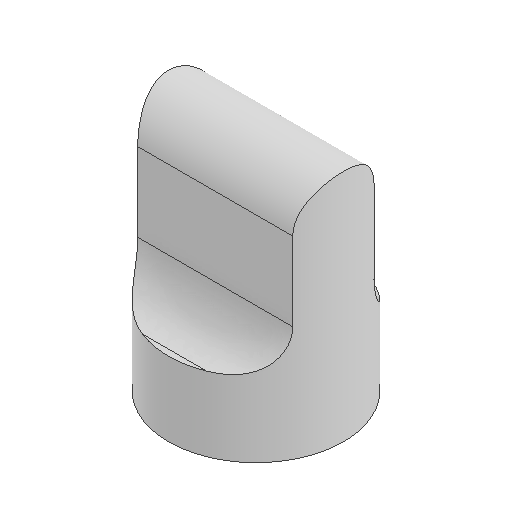
# Autodesk Inventor part: Half Universal
Saved by Autodesk Inventor 2025 (Build 290162010, 162A)
## iProperties
Created: 2024-12-02
Part Number: Half Universal
Material: Generic
Document SubType Name: Modeling
Designer: ALEXANDERNICHOLS
Density: 1 g/cm^3
Appearance: Default
Author: ALEXANDERNICHOLS
Autodesk Inventor part; units mm, degrees
ref_plane "YZ Plane" through (0, 0, 0) normal (1, 0, 0) x (0, 1, 0)
ref_plane "XZ Plane" through (0, 0, 0) normal (0, 1, 0) x (-1, 0, 0)
ref_plane "XY Plane" through (0, 0, 0) normal (0, 0, 1) x (1, 0, 0)
sketch "Sketch1" plane through (0, 0, 0) normal (0, 1, 0) x (-1, 0, 0)
  circle A0 centre (0, 0) radius 2.54
  circle A1 centre (0, 0) radius 5.461
  dimension "d0" = 5.08
  dimension "d1" = 10.922
  constraints: 2 centre point, 2 coincident
  measures "d0" diameter of A0
  measures "d1" diameter of A1
extrude "Extrusion1" add sketch "Sketch1" along normal blind 14.605 contours A0 | A1
sketch "Sketch2" plane through (0, 0, 0) normal (1, 0, 0) x (0, 1, 0)
  arc A0 (12.065, -2.54) -> (12.065, 2.54) centre (12.065, 0) ccw
  line L0 (0, 5.461) -> (14.605, 5.461) projected
  line L1 (0, -5.461) -> (14.605, -5.461) projected
  line L2 (12.065, 2.54) -> (7.1656, 2.54)
  line L3 (12.065, -2.54) -> (7.1656, -2.54)
  line L4 (4.6256, 5.461) -> (4.6256, 5.08)
  line L5 (4.6256, -5.08) -> (4.6256, -5.461)
  arc A1 (4.6256, 5.08) -> (7.1656, 2.54) centre (7.1656, 5.08) ccw
  arc A2 (7.1656, -2.54) -> (4.6256, -5.08) centre (7.1656, -5.08) ccw
  line L6 (14.605, 2.54) -> (14.605, -2.54) projected
  line L7 (14.605, -5.461) -> (14.605, 5.461) projected
  point P0 (0, 0)
  point P1 (14.605, 0)
  dimension "d4" = 2.54
  dimension "d5" = 2.54
  constraints: 8 end point, 7 tangent, 6 perpendicular, 6 point on circle, 3 centre point, 2 point on line, 1 equal radius
  measures "d4" radius of A1
  measures "d5" radius of A0
extrude "Extrusion2" cut sketch "Sketch2" along normal mid plane 14.605
body "Solid1"
